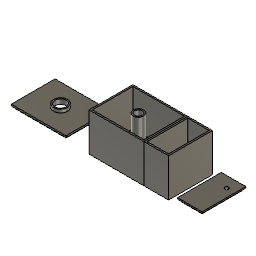
atomizer_v1 (Autodesk Fusion 360 design; units mm, degrees)
part number: 2026-08-18-11-35-30-436
Autodesk Fusion 360 part; units mm, degrees
sketch "Sketch1" plane through (0, 0, 0) normal (0, 0, 1) x (1, 0, 0)
  line L0 (0, 0) -> (100, 0)
  line L1 (100, 0) -> (100, 80)
  line L2 (100, 80) -> (0, 80)
  line L3 (0, 80) -> (0, 0)
sketch "Sketch2" plane through (0, 0, 0) normal (0, 0, 1) x (1, 0, 0)
  line L0 (100, 0) -> (145, 0)
  line L1 (145, 0) -> (145, 80)
  line L2 (145, 80) -> (100, 80)
  line L3 (100, 80) -> (100, 0)
sketch "Sketch3" plane through (0, 0, 0) normal (0, 0, 1) x (1, 0, 0)
  line L0 (3, 3) -> (97, 3)
  line L1 (97, 3) -> (97, 77)
  line L2 (97, 77) -> (3, 77)
  line L3 (3, 77) -> (3, 3)
sketch "Sketch4" plane through (0, 0, 0) normal (0, 0, 1) x (1, 0, 0)
  line L0 (103, 3) -> (142, 3)
  line L1 (142, 3) -> (142, 77)
  line L2 (142, 77) -> (103, 77)
  line L3 (103, 77) -> (103, 3)
sketch "Sketch5" plane through (0, 0, 0) normal (0, 0, 1) x (1, 0, 0)
  line L0 (0, 0) -> (100, 0)
  line L1 (100, 0) -> (100, 80)
  line L2 (100, 80) -> (0, 80)
  line L3 (0, 80) -> (0, 0)
extrude "Extrude5" add sketch "Sketch5" along normal blind 70 makes body 1
shell "Shell1" thickness 3 removed faces 1 at (33.3333, 53.3333, 70) on bodies 1
sketch "Sketch6" plane through (0, 0, 0) normal (0, 0, 1) x (1, 0, 0)
  line L0 (100, 0) -> (145, 0)
  line L1 (145, 0) -> (145, 80)
  line L2 (145, 80) -> (100, 80)
  line L3 (100, 80) -> (100, 0)
extrude "Extrude6" add sketch "Sketch6" along normal blind 70 separate body makes body 2
shell "Shell2" thickness 3 removed faces 1 at (115, 53.3333, 70) on bodies 2
sketch "Sketch7" plane through (0, 0, 0) normal (0, 0, 1) x (1, 0, 0)
  line L0 (100, 0) -> (145, 0)
  line L1 (145, 0) -> (145, 80)
  line L2 (145, 80) -> (100, 80)
  line L3 (100, 80) -> (100, 0)
extrude "Extrude7" add sketch "Sketch7" along normal blind 2.5 from surface at 70 separate body makes body 3
sketch "Sketch8" plane through (0, 0, 0) normal (0, 0, 1) x (1, 0, 0)
  line L0 (103.3, 3.3) -> (141.7, 3.3)
  line L1 (141.7, 3.3) -> (141.7, 76.7)
  line L2 (141.7, 76.7) -> (103.3, 76.7)
  line L3 (103.3, 76.7) -> (103.3, 3.3)
extrude "Extrude8" add sketch "Sketch8" along normal blind 4 from surface at 66 bodies 3
sketch "Sketch9" plane through (0, 0, 0) normal (0, 0, 1) x (1, 0, 0)
  line L0 (105.3, 5.3) -> (139.7, 5.3)
  line L1 (139.7, 5.3) -> (139.7, 74.7)
  line L2 (139.7, 74.7) -> (105.3, 74.7)
  line L3 (105.3, 74.7) -> (105.3, 5.3)
extrude "Extrude9" cut sketch "Sketch9" along normal blind 4 from surface at 66 bodies 3
sketch "Sketch10" plane through (0, 0, 0) normal (0, 0, 1) x (1, 0, 0)
  circle A0 centre (130, 60) radius 3.5
extrude "Extrude10" cut sketch "Sketch10" along normal blind 2.5 from surface at 70 bodies 3
sketch "Sketch11" plane through (0, 0, 0) normal (0, 0, 1) x (1, 0, 0)
  line L0 (0, 0) -> (100, 0)
  line L1 (100, 0) -> (100, 80)
  line L2 (100, 80) -> (0, 80)
  line L3 (0, 80) -> (0, 0)
extrude "Extrude11" add sketch "Sketch11" along normal blind 3 from surface at 70 separate body makes body 4
sketch "Sketch12" plane through (0, 0, 0) normal (0, 0, 1) x (1, 0, 0)
  line L0 (3.3, 3.3) -> (96.7, 3.3)
  line L1 (96.7, 3.3) -> (96.7, 76.7)
  line L2 (96.7, 76.7) -> (3.3, 76.7)
  line L3 (3.3, 76.7) -> (3.3, 3.3)
extrude "Extrude12" add sketch "Sketch12" along normal blind 4 from surface at 66 bodies 4
sketch "Sketch13" plane through (0, 0, 0) normal (0, 0, 1) x (1, 0, 0)
  line L0 (5.3, 5.3) -> (94.7, 5.3)
  line L1 (94.7, 5.3) -> (94.7, 74.7)
  line L2 (94.7, 74.7) -> (5.3, 74.7)
  line L3 (5.3, 74.7) -> (5.3, 5.3)
extrude "Extrude13" cut sketch "Sketch13" along normal blind 4 from surface at 66 bodies 4
sketch "Sketch14" plane through (0, 0, 0) normal (0, 0, 1) x (1, 0, 0)
  circle A0 centre (50, 40) radius 12.7
extrude "Extrude14" add sketch "Sketch14" along normal blind 6 from surface at 73 bodies 4
sketch "Sketch15" plane through (0, 0, 0) normal (0, 0, 1) x (1, 0, 0)
  circle A0 centre (50, 40) radius 10.2
extrude "Extrude15" cut sketch "Sketch15" along normal blind 6 from surface at 73 bodies 4
sketch "Sketch16" plane through (0, 0, 0) normal (0, 0, 1) x (1, 0, 0)
  circle A0 centre (50, 40) radius 10.2
extrude "Extrude16" cut sketch "Sketch16" along normal blind 3 from surface at 70 bodies 4
sketch "Sketch17" plane through (0, 0, 0) normal (0, 0, 1) x (1, 0, 0)
  circle A0 centre (50, 40) radius 9.5
sketch "Sketch18" plane through (0, 0, 0) normal (0, 0, 1) x (1, 0, 0)
  circle A0 centre (50, 40) radius 7
sketch "Sketch19" plane through (0, 0, 0) normal (0, 0, 1) x (1, 0, 0)
  line L0 (48, 47) -> (52, 47)
  line L1 (52, 47) -> (52, 49.5)
  line L2 (52, 49.5) -> (48, 49.5)
  line L3 (48, 49.5) -> (48, 47)
sketch "Sketch20" plane through (0, 0, 0) normal (0, 0, 1) x (1, 0, 0)
  line L0 (48, 30.5) -> (52, 30.5)
  line L1 (52, 30.5) -> (52, 33)
  line L2 (52, 33) -> (48, 33)
  line L3 (48, 33) -> (48, 30.5)
sketch "Sketch21" plane through (0, 0, 0) normal (0, 0, 1) x (1, 0, 0)
  line L0 (57, 38) -> (59.5, 38)
  line L1 (59.5, 38) -> (59.5, 42)
  line L2 (59.5, 42) -> (57, 42)
  line L3 (57, 42) -> (57, 38)
sketch "Sketch22" plane through (0, 0, 0) normal (0, 0, 1) x (1, 0, 0)
  line L0 (40.5, 38) -> (43, 38)
  line L1 (43, 38) -> (43, 42)
  line L2 (43, 42) -> (40.5, 42)
  line L3 (40.5, 42) -> (40.5, 38)
sketch "Sketch23" plane through (0, 0, 0) normal (0, 0, 1) x (1, 0, 0)
  circle A0 centre (50, 40) radius 9.5
sketch "Sketch24" plane through (0, 0, 0) normal (0, 0, 1) x (1, 0, 0)
  circle A0 centre (50, 40) radius 7
sketch "Sketch25" plane through (0, 0, 0) normal (0, 0, 1) x (1, 0, 0)
  line L0 (48, 47) -> (52, 47)
  line L1 (52, 47) -> (52, 49.5)
  line L2 (52, 49.5) -> (48, 49.5)
  line L3 (48, 49.5) -> (48, 47)
sketch "Sketch29" plane through (0, 0, 0) normal (0, 0, 1) x (1, 0, 0)
  circle A0 centre (50, 40) radius 9.5
extrude "Extrude29" add sketch "Sketch29" along normal blind 66 from surface at 4 separate body makes body 5
sketch "Sketch30" plane through (0, 0, 0) normal (0, 0, 1) x (1, 0, 0)
  circle A0 centre (50, 40) radius 7
extrude "Extrude30" cut sketch "Sketch30" along normal blind 66 from surface at 4 bodies 5
sketch "Sketch31" plane through (0, 0, 0) normal (0, 0, 1) x (1, 0, 0)
  line L0 (48, 47) -> (52, 47)
  line L1 (52, 47) -> (52, 49.5)
  line L2 (52, 49.5) -> (48, 49.5)
  line L3 (48, 49.5) -> (48, 47)
extrude "Extrude31" cut sketch "Sketch31" along normal blind 10 from surface at 7 bodies 5
sketch "Sketch32" plane through (0, 0, 0) normal (0, 0, 1) x (1, 0, 0)
  line L0 (48, 30.5) -> (52, 30.5)
  line L1 (52, 30.5) -> (52, 33)
  line L2 (52, 33) -> (48, 33)
  line L3 (48, 33) -> (48, 30.5)
extrude "Extrude32" cut sketch "Sketch32" along normal blind 10 from surface at 7 bodies 5
sketch "Sketch33" plane through (0, 0, 0) normal (0, 0, 1) x (1, 0, 0)
  line L0 (57, 38) -> (59.5, 38)
  line L1 (59.5, 38) -> (59.5, 42)
  line L2 (59.5, 42) -> (57, 42)
  line L3 (57, 42) -> (57, 38)
extrude "Extrude33" cut sketch "Sketch33" along normal blind 10 from surface at 7 bodies 5
sketch "Sketch34" plane through (0, 0, 0) normal (0, 0, 1) x (1, 0, 0)
  line L0 (40.5, 38) -> (43, 38)
  line L1 (43, 38) -> (43, 42)
  line L2 (43, 42) -> (40.5, 42)
  line L3 (40.5, 42) -> (40.5, 38)
extrude "Extrude34" cut sketch "Sketch34" along normal blind 10 from surface at 7 bodies 5
move_body "Move29" bodies 4 to x (1, 0, 0) y (0, 1, 0) z (0, 0, 1) at (-143.9651, 2.1058, -66.9438)
move_body "Move30" bodies 3 to x (1, 0, 0) y (0, 1, 0) z (0, 0, 1) at (56.3198, 4.7558, -65.1575)
named bodies: "WaterReservoir", "Electronics", "Lid_Electronics", "Lid_WaterReservoir", "WickGuide"
